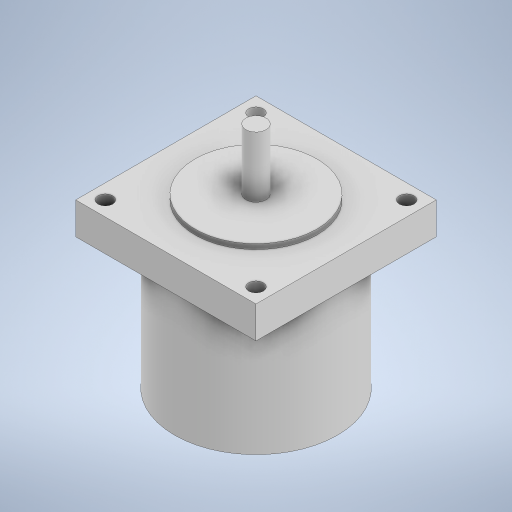
# Autodesk Inventor part: Motor model
Saved by Autodesk Inventor 2023 (Build 270158000, 158)
## iProperties
Created: 2023-02-22
Part Number: Motor model
Material: Generic
Document SubType Name: Modeling
Designer: cheng
Density: 1 g/cm^3
Appearance: Default
Author: cheng
Autodesk Inventor part; units mm, degrees
ref_plane "YZ Plane" through (0, 0, 0) normal (1, 0, 0) x (0, 1, 0)
ref_plane "XZ Plane" through (0, 0, 0) normal (0, 1, 0) x (-1, 0, 0)
ref_plane "XY Plane" through (0, 0, 0) normal (0, 0, 1) x (1, 0, 0)
sketch "Sketch1" plane through (0, 0, 0) normal (0, 1, 0) x (-1, 0, 0)
  line L0 (28.2, 28.2) -> (-28.2, 28.2)
  line L1 (-28.2, 28.2) -> (-28.2, -28.2)
  line L2 (-28.2, -28.2) -> (28.2, -28.2)
  line L3 (28.2, -28.2) -> (28.2, 28.2)
  line L4 (28.2, 28.2) -> (-28.2, -28.2) construction
  line L5 (-28.2, 28.2) -> (28.2, -28.2) construction
  line L6 (0, 28.2) -> (0, -28.2) construction
  line L7 (28.2, 0) -> (-28.2, 0) construction
  circle A0 centre (23.57, 23.57) radius 2.3
  circle A1 centre (23.57, -23.57) radius 2.3
  circle A2 centre (-23.57, 23.57) radius 2.3
  circle A3 centre (-23.57, -23.57) radius 2.3
  point P0 (0, 0)
  dimension "d0" = 56.4
  dimension "d1" = 56.4
  dimension "d2" = 4.6
  dimension "d5" = 47.14
  dimension "d6" = 47.14
  constraints: 16 end point, 6 midpoint, 4 centre point, 3 symmetric about line, 2 parallel, 1 horizontal, 1 perpendicular, 3 other
  measures "d0" distance of L2.end L0.start
  measures "d1" distance between parallel lines of L1 L3
  measures "d2" diameter of A0
  measures "d5" distance of A1.centre A0.centre
  measures "d6" distance of A2.centre A0.centre
extrude "Extrusion1" add sketch "Sketch1" along normal blind 10
sketch "Sketch2" plane through (0, 0, 0) normal (0, -1, 0) x (1, 0, 0)
  circle A0 centre (0, 0) radius 25.5
  dimension "d9" = 51
  constraints: 1 centre point, 1 coincident
  measures "d9" diameter of A0
extrude "Extrusion2" add sketch "Sketch2" along normal blind 41
sketch "Sketch3" plane through (0, 10, 0) normal (0, 1, 0) x (1, 0, 0)
  circle A0 centre (0, 0) radius 19.05
  dimension "d12" = 38.1
  constraints: 1 centre point, 1 coincident
  measures "d12" diameter of A0
extrude "Extrusion3" add sketch "Sketch3" along normal blind 1.6
sketch "Sketch4" plane through (0, 11.6, 0) normal (0, 1, 0) x (1, 0, 0)
  circle A0 centre (0, 0) radius 3.175
  dimension "d15" = 6.35
  constraints: 1 centre point, 1 coincident
  measures "d15" diameter of A0
extrude "Extrusion4" add sketch "Sketch4" along normal blind 19
body "Solid1"
